Autodesk Fusion 360 part; units mm, degrees
note: some values were not read from the file. Set by a fixed rule: which sketch regions a step uses.
(part 4 of 6)
  spline S14 degree 5 poles (-6.3022, 4.9084) (-6.3022, 4.9084) (-6.3024, 4.9085) (-6.3026, 4.9086) (-6.3029, 4.9089) (-6.3033, 4.9092) (-6.3039, 4.9096) (-6.3045, 4.9101) (-6.3052, 4.9106) (-6.3059, 4.9111) (-6.3067, 4.9117) (-6.3076, 4.9124) (-6.3086, 4.913) (-6.3096, 4.9138) (-6.3107, 4.9145) (-6.3119, 4.9153) (-6.3131, 4.9162) (-6.3144, 4.9171) (-6.3158, 4.918) (-6.3173, 4.919) (-6.3188, 4.92) (-6.3203, 4.9211) (-6.322, 4.9221) (-6.3237, 4.9233) (-6.3254, 4.9244) (-6.3273, 4.9256) (-6.3292, 4.9268) (-6.3311, 4.9281) (-6.3332, 4.9294) (-6.3353, 4.9307) (-6.3374, 4.932) (-6.3396, 4.9334) (-6.3419, 4.9348) (-6.3443, 4.9363) (-6.3467, 4.9377) (-6.3491, 4.9392) (-6.3517, 4.9407) (-6.3543, 4.9423) (-6.3569, 4.9439) (-6.3596, 4.9454) (-6.3624, 4.9471) (-6.3652, 4.9487) (-6.3681, 4.9504) (-6.3711, 4.9521) (-6.3741, 4.9538) (-6.3772, 4.9555) (-6.3803, 4.9573) (-6.3835, 4.9591) (-6.3868, 4.9608) (-6.3901, 4.9627) (-6.3934, 4.9645) (-6.3969, 4.9664) (-6.4003, 4.9682) (-6.4039, 4.9701) (-6.4075, 4.972) (-6.4111, 4.9739) (-6.4149, 4.9759) (-6.4186, 4.9778) (-6.4224, 4.9798) (-6.4263, 4.9818) (-6.4303, 4.9838) (-6.4343, 4.9858) (-6.4383, 4.9878) (-6.4424, 4.9899) (-6.4466, 4.9919) (-6.4508, 4.994) (-6.455, 4.9961) (-6.4594, 4.9981) (-6.4637, 5.0002) (-6.4682, 5.0023) (-6.4727, 5.0045) (-6.4772, 5.0066) (-6.4818, 5.0087) (-6.4864, 5.0109) (-6.4911, 5.013) (-6.4959, 5.0152) (-6.5007, 5.0174) (-6.5055, 5.0195) (-6.5104, 5.0217) (-6.5154, 5.0239) (-6.5204, 5.0261) (-6.5255, 5.0283) (-6.5306, 5.0305) (-6.5357, 5.0327) (-6.541, 5.0349) (-6.5462, 5.0372) (-6.5515, 5.0394) (-6.5569, 5.0416) (-6.5623, 5.0439) (-6.5678, 5.0461) (-6.5733, 5.0483) (-6.5789, 5.0506) (-6.5845, 5.0528) (-6.5901, 5.0551) (-6.5959, 5.0573) (-6.6016, 5.0596) (-6.6074, 5.0618) (-6.6133, 5.0641) (-6.6192, 5.0664) (-6.6252, 5.0686) (-6.6312, 5.0709) (-6.6372, 5.0731) (-6.6433, 5.0754) (-6.6495, 5.0776) (-6.6556, 5.0799) (-6.6619, 5.0821) (-6.6682, 5.0844) (-6.6745, 5.0866) (-6.6809, 5.0889) (-6.6873, 5.0911) (-6.6938, 5.0933) (-6.7003, 5.0956) (-6.7069, 5.0978) (-6.7135, 5.1) (-6.7201, 5.1023) (-6.7269, 5.1045) (-6.7336, 5.1067) (-6.7404, 5.1089) (-6.7472, 5.1111) (-6.7541, 5.1133) (-6.761, 5.1155) (-6.768, 5.1177) (-6.775, 5.1199) (-6.7821, 5.1221) (-6.7892, 5.1242) (-6.7963, 5.1264) (-6.8035, 5.1286) (-6.8108, 5.1307) (-6.818, 5.1329) (-6.8254, 5.135) (-6.8327, 5.1371) (-6.8401, 5.1393) (-6.8476, 5.1414) (-6.8551, 5.1435) (-6.8626, 5.1456) (-6.8702, 5.1477) (-6.8778, 5.1498) (-6.8855, 5.1518) (-6.8932, 5.1539) (-6.9009, 5.1559) (-6.9087, 5.158) (-6.9165, 5.16) (-6.9244, 5.162) (-6.9323, 5.164) (-6.9403, 5.166) (-6.9483, 5.168) (-6.9563, 5.17) (-6.9644, 5.172) (-6.9725, 5.1739) (-6.9806, 5.1759) (-6.9888, 5.1778) (-6.997, 5.1797) (-7.0053, 5.1817) (-7.0136, 5.1836) (-7.022, 5.1854) (-7.0304, 5.1873) (-7.0388, 5.1892) (-7.0473, 5.191) (-7.0558, 5.1929) (-7.0643, 5.1947) (-7.0729, 5.1965) (-7.0815, 5.1983) (-7.0902, 5.2001) (-7.0989, 5.2018) (-7.1076, 5.2036) (-7.1164, 5.2053) (-7.1252, 5.207) (-7.1341, 5.2087) (-7.1429, 5.2104) (-7.1519, 5.2121) (-7.1608, 5.2138) (-7.1698, 5.2154) (-7.1789, 5.2171) (-7.1879, 5.2187) (-7.197, 5.2203) (-7.2062, 5.2219) (-7.2154, 5.2234) (-7.2246, 5.225) (-7.2338, 5.2265) (-7.2431, 5.228) (-7.2524, 5.2295) (-7.2618, 5.231) (-7.2712, 5.2325) (-7.2806, 5.2339) (-7.2901, 5.2354) (-7.2996, 5.2368) (-7.3091, 5.2382) (-7.3187, 5.2396) (-7.3283, 5.2409) (-7.3379, 5.2423) (-7.3476, 5.2436) (-7.3573, 5.2449) (-7.3671, 5.2462) (-7.3768, 5.2475) (-7.3866, 5.2487) (-7.3965, 5.25) (-7.4064, 5.2512) (-7.4163, 5.2524) (-7.4262, 5.2536) (-7.4362, 5.2547) (-7.4462, 5.2559) (-7.4562, 5.257) (-7.4663, 5.2581) (-7.4764, 5.2592) (-7.4865, 5.2602) (-7.4967, 5.2613) (-7.5069, 5.2623) (-7.5172, 5.2633) (-7.5274, 5.2642) (-7.5377, 5.2652) (-7.5481, 5.2661) (-7.5584, 5.2671) (-7.5688, 5.2679) (-7.5792, 5.2688) (-7.5897, 5.2697) (-7.6002, 5.2705) (-7.6107, 5.2713) (-7.6212, 5.2721) (-7.6318, 5.2729) (-7.6424, 5.2736) (-7.6531, 5.2743) (-7.6637, 5.275) (-7.6744, 5.2757) (-7.6852, 5.2764) (-7.6959, 5.277) (-7.7067, 5.2776) (-7.7175, 5.2782) (-7.7284, 5.2788) (-7.7393, 5.2793) (-7.7502, 5.2798) (-7.7611, 5.2803) (-7.7721, 5.2808) (-7.7831, 5.2813) (-7.7941, 5.2817) (-7.8052, 5.2821) (-7.8162, 5.2825) (-7.8273, 5.2828) (-7.8385, 5.2832) (-7.8496, 5.2835) (-7.8608, 5.2837) (-7.8721, 5.284) (-7.8811, 5.2842) (-7.8878, 5.2843) (-7.8923, 5.2844) (-7.8946, 5.2845) knots 0 0 0 0 0 0 0.00416667 0.00833333 0.0125 0.01666667 0.02083333 0.025 0.02916667 0.03333333 0.0375 0.04166667 0.04583333 0.05 0.05416667 0.05833333 0.0625 0.06666667 0.07083333 0.075 0.07916667 0.08333333 0.0875 0.09166667 0.09583333 0.1 0.10416667 0.10833333 0.1125 0.11666667 0.12083333 0.125 0.12916667 0.13333333 0.1375 0.14166667 0.14583333 0.15 0.15416667 0.15833333 0.1625 0.16666667 0.17083333 0.175 0.17916667 0.18333333 0.1875 0.19166667 0.19583333 0.2 0.20416667 0.20833333 0.2125 0.21666667 0.22083333 0.225 0.22916667 0.23333333 0.2375 0.24166667 0.24583333 0.25 0.25416667 0.25833333 0.2625 0.26666667 0.27083333 0.275 0.27916667 0.28333333 0.2875 0.29166667 0.29583333 0.3 0.30416667 0.30833333 0.3125 0.31666667 0.32083333 0.325 0.32916667 0.33333333 0.3375 0.34166667 0.34583333 0.35 0.35416667 0.35833333 0.3625 0.36666667 0.37083333 0.375 0.37916667 0.38333333 0.3875 0.39166667 0.39583333 0.4 0.40416667 0.40833333 0.4125 0.41666667 0.42083333 0.425 0.42916667 0.43333333 0.4375 0.44166667 0.44583333 0.45 0.45416667 0.45833333 0.4625 0.46666667 0.47083333 0.475 0.47916667 0.48333333 0.4875 0.49166667 0.49583333 0.5 0.50416667 0.50833333 0.5125 0.51666667 0.52083333 0.525 0.52916667 0.53333333 0.5375 0.54166667 0.54583333 0.55 0.55416667 0.55833333 0.5625 0.56666667 0.57083333 0.575 0.57916667 0.58333333 0.5875 0.59166667 0.59583333 0.6 0.60416667 0.60833333 0.6125 0.61666667 0.62083333 0.625 0.62916667 0.63333333 0.6375 0.64166667 0.64583333 0.65 0.65416667 0.65833333 0.6625 0.66666667 0.67083333 0.675 0.67916667 0.68333333 0.6875 0.69166667 0.69583333 0.7 0.70416667 0.70833333 0.7125 0.71666667 0.72083333 0.725 0.72916667 0.73333333 0.7375 0.74166667 0.74583333 0.75 0.75416667 0.75833333 0.7625 0.76666667 0.77083333 0.775 0.77916667 0.78333333 0.7875 0.79166667 0.79583333 0.8 0.80416667 0.80833333 0.8125 0.81666667 0.82083333 0.825 0.82916667 0.83333333 0.8375 0.84166667 0.84583333 0.85 0.85416667 0.85833333 0.8625 0.86666667 0.87083333 0.875 0.87916667 0.88333333 0.8875 0.89166667 0.89583333 0.9 0.90416667 0.90833333 0.9125 0.91666667 0.92083333 0.925 0.92916667 0.93333333 0.9375 0.94166667 0.94583333 0.95 0.95416667 0.95833333 0.9625 0.96666667 0.97083333 0.975 0.97916667 0.98333333 0.9875 0.99166667 0.99583333 1 1 1 1 1 1
  arc A15 (-7.8946, 5.2845) -> (-8.2494, 4.7115) centre (0, 0) ccw
  spline S15 degree 5 poles (-8.2494, 4.7115) (-8.2483, 4.7095) (-8.2462, 4.7055) (-8.2431, 4.6995) (-8.2389, 4.6915) (-8.2337, 4.6816) (-8.2284, 4.6717) (-8.2232, 4.6618) (-8.2179, 4.652) (-8.2127, 4.6422) (-8.2074, 4.6325) (-8.2021, 4.6227) (-8.1968, 4.6131) (-8.1915, 4.6034) (-8.1862, 4.5938) (-8.1809, 4.5843) (-8.1755, 4.5747) (-8.1702, 4.5652) (-8.1649, 4.5558) (-8.1595, 4.5463) (-8.1542, 4.537) (-8.1488, 4.5276) (-8.1434, 4.5183) (-8.138, 4.509) (-8.1327, 4.4998) (-8.1273, 4.4906) (-8.1219, 4.4814) (-8.1165, 4.4723) (-8.1111, 4.4632) (-8.1057, 4.4541) (-8.1002, 4.4451) (-8.0948, 4.4361) (-8.0894, 4.4272) (-8.084, 4.4183) (-8.0785, 4.4094) (-8.0731, 4.4006) (-8.0676, 4.3918) (-8.0622, 4.383) (-8.0567, 4.3743) (-8.0513, 4.3656) (-8.0458, 4.357) (-8.0403, 4.3484) (-8.0349, 4.3398) (-8.0294, 4.3313) (-8.0239, 4.3228) (-8.0184, 4.3144) (-8.0129, 4.306) (-8.0075, 4.2976) (-8.002, 4.2892) (-7.9965, 4.2809) (-7.991, 4.2727) (-7.9855, 4.2645) (-7.98, 4.2563) (-7.9745, 4.2481) (-7.969, 4.24) (-7.9635, 4.232) (-7.958, 4.2239) (-7.9525, 4.2159) (-7.947, 4.208) (-7.9415, 4.2001) (-7.936, 4.1922) (-7.9305, 4.1844) (-7.925, 4.1766) (-7.9195, 4.1688) (-7.914, 4.1611) (-7.9085, 4.1534) (-7.903, 4.1458) (-7.8975, 4.1382) (-7.892, 4.1306) (-7.8865, 4.1231) (-7.881, 4.1156) (-7.8755, 4.1082) (-7.87, 4.1008) (-7.8645, 4.0934) (-7.859, 4.0861) (-7.8536, 4.0788) (-7.8481, 4.0716) (-7.8426, 4.0644) (-7.8371, 4.0572) (-7.8317, 4.0501) (-7.8262, 4.043) (-7.8207, 4.036) (-7.8153, 4.029) (-7.8098, 4.022) (-7.8044, 4.0151) (-7.7989, 4.0082) (-7.7935, 4.0014) (-7.788, 3.9946) (-7.7826, 3.9879) (-7.7772, 3.9811) (-7.7718, 3.9745) (-7.7664, 3.9678) (-7.761, 3.9612) (-7.7556, 3.9547) (-7.7502, 3.9482) (-7.7448, 3.9417) (-7.7394, 3.9353) (-7.7341, 3.9289) (-7.7287, 3.9225) (-7.7233, 3.9162) (-7.718, 3.91) (-7.7127, 3.9037) (-7.7073, 3.8976) (-7.702, 3.8914) (-7.6967, 3.8853) (-7.6914, 3.8793) (-7.6861, 3.8732) (-7.6808, 3.8673) (-7.6756, 3.8613) (-7.6703, 3.8554) (-7.6651, 3.8496) (-7.6598, 3.8438) (-7.6546, 3.838) (-7.6494, 3.8323) (-7.6442, 3.8266) (-7.639, 3.8209) (-7.6338, 3.8153) (-7.6287, 3.8098) (-7.6235, 3.8043) (-7.6184, 3.7988) (-7.6132, 3.7934) (-7.6081, 3.788) (-7.603, 3.7826) (-7.5979, 3.7773) (-7.5929, 3.7721) (-7.5878, 3.7668) (-7.5828, 3.7616) (-7.5778, 3.7565) (-7.5728, 3.7514) (-7.5678, 3.7464) (-7.5628, 3.7414) (-7.5578, 3.7364) (-7.5529, 3.7315) (-7.548, 3.7266) (-7.5431, 3.7217) (-7.5382, 3.7169) (-7.5333, 3.7122) (-7.5284, 3.7075) (-7.5236, 3.7028) (-7.5188, 3.6982) (-7.514, 3.6936) (-7.5092, 3.6891) (-7.5045, 3.6846) (-7.4997, 3.6801) (-7.495, 3.6757) (-7.4903, 3.6713) (-7.4856, 3.667) (-7.481, 3.6627) (-7.4764, 3.6585) (-7.4718, 3.6543) (-7.4672, 3.6501) (-7.4626, 3.646) (-7.4581, 3.6419) (-7.4536, 3.6379) (-7.4491, 3.6339) (-7.4446, 3.63) (-7.4402, 3.6261) (-7.4357, 3.6222) (-7.4314, 3.6184) (-7.427, 3.6147) (-7.4227, 3.611) (-7.4183, 3.6073) (-7.4141, 3.6036) (-7.4098, 3.6) (-7.4056, 3.5965) (-7.4014, 3.593) (-7.3972, 3.5895) (-7.3931, 3.5861) (-7.389, 3.5827) (-7.3849, 3.5794) (-7.3808, 3.5761) (-7.3768, 3.5729) (-7.3728, 3.5697) (-7.3688, 3.5665) (-7.3649, 3.5634) (-7.361, 3.5603) (-7.3572, 3.5573) (-7.3533, 3.5543) (-7.3495, 3.5514) (-7.3458, 3.5485) (-7.3421, 3.5456) (-7.3384, 3.5428) (-7.3347, 3.5401) (-7.3311, 3.5374) (-7.3275, 3.5347) (-7.324, 3.532) (-7.3205, 3.5295) (-7.317, 3.5269) (-7.3136, 3.5244) (-7.3102, 3.5219) (-7.3068, 3.5195) (-7.3035, 3.5172) (-7.3003, 3.5148) (-7.297, 3.5125) (-7.2938, 3.5103) (-7.2907, 3.5081) (-7.2876, 3.506) (-7.2845, 3.5038) (-7.2815, 3.5018) (-7.2786, 3.4998) (-7.2756, 3.4978) (-7.2728, 3.4958) (-7.2699, 3.4939) (-7.2671, 3.4921) (-7.2644, 3.4903) (-7.2617, 3.4885) (-7.2591, 3.4868) (-7.2565, 3.4851) (-7.2539, 3.4835) (-7.2515, 3.4819) (-7.249, 3.4804) (-7.2466, 3.4789) (-7.2443, 3.4774) (-7.242, 3.476) (-7.2398, 3.4746) (-7.2376, 3.4733) (-7.2355, 3.472) (-7.2335, 3.4708) (-7.2315, 3.4696) (-7.2295, 3.4684) (-7.2276, 3.4673) (-7.2258, 3.4662) (-7.2241, 3.4652) (-7.2224, 3.4642) (-7.2207, 3.4633) (-7.2191, 3.4624) (-7.2176, 3.4615) (-7.2162, 3.4607) (-7.2148, 3.46) (-7.2135, 3.4592) (-7.2122, 3.4585) (-7.2111, 3.4579) (-7.21, 3.4573) (-7.2089, 3.4567) (-7.2079, 3.4562) (-7.207, 3.4558) (-7.2062, 3.4553) (-7.2055, 3.4549) (-7.2048, 3.4546) (-7.2042, 3.4543) (-7.2037, 3.454) (-7.2033, 3.4538) (-7.2031, 3.4537) (-7.203, 3.4537) (-7.2029, 3.4536) knots -1 -1 -1 -1 -1 -1 -0.99583333 -0.99166667 -0.9875 -0.98333333 -0.97916667 -0.975 -0.97083333 -0.96666667 -0.9625 -0.95833333 -0.95416667 -0.95 -0.94583333 -0.94166667 -0.9375 -0.93333333 -0.92916667 -0.925 -0.92083333 -0.91666667 -0.9125 -0.90833333 -0.90416667 -0.9 -0.89583333 -0.89166667 -0.8875 -0.88333333 -0.87916667 -0.875 -0.87083333 -0.86666667 -0.8625 -0.85833333 -0.85416667 -0.85 -0.84583333 -0.84166667 -0.8375 -0.83333333 -0.82916667 -0.825 -0.82083333 -0.81666667 -0.8125 -0.80833333 -0.80416667 -0.8 -0.79583333 -0.79166667 -0.7875 -0.78333333 -0.77916667 -0.775 -0.77083333 -0.76666667 -0.7625 -0.75833333 -0.75416667 -0.75 -0.74583333 -0.74166667 -0.7375 -0.73333333 -0.72916667 -0.725 -0.72083333 -0.71666667 -0.7125 -0.70833333 -0.70416667 -0.7 -0.69583333 -0.69166667 -0.6875 -0.68333333 -0.67916667 -0.675 -0.67083333 -0.66666667 -0.6625 -0.65833333 -0.65416667 -0.65 -0.64583333 -0.64166667 -0.6375 -0.63333333 -0.62916667 -0.625 -0.62083333 -0.61666667 -0.6125 -0.60833333 -0.60416667 -0.6 -0.59583333 -0.59166667 -0.5875 -0.58333333 -0.57916667 -0.575 -0.57083333 -0.56666667 -0.5625 -0.55833333 -0.55416667 -0.55 -0.54583333 -0.54166667 -0.5375 -0.53333333 -0.52916667 -0.525 -0.52083333 -0.51666667 -0.5125 -0.50833333 -0.50416667 -0.5 -0.49583333 -0.49166667 -0.4875 -0.48333333 -0.47916667 -0.475 -0.47083333 -0.46666667 -0.4625 -0.45833333 -0.45416667 -0.45 -0.44583333 -0.44166667 -0.4375 -0.43333333 -0.42916667 -0.425 -0.42083333 -0.41666667 -0.4125 -0.40833333 -0.40416667 -0.4 -0.39583333 -0.39166667 -0.3875 -0.38333333 -0.37916667 -0.375 -0.37083333 -0.36666667 -0.3625 -0.35833333 -0.35416667 -0.35 -0.34583333 -0.34166667 -0.3375 -0.33333333 -0.32916667 -0.325 -0.32083333 -0.31666667 -0.3125 -0.30833333 -0.30416667 -0.3 -0.29583333 -0.29166667 -0.2875 -0.28333333 -0.27916667 -0.275 -0.27083333 -0.26666667 -0.2625 -0.25833333 -0.25416667 -0.25 -0.24583333 -0.24166667 -0.2375 -0.23333333 -0.22916667 -0.225 -0.22083333 -0.21666667 -0.2125 -0.20833333 -0.20416667 -0.2 -0.19583333 -0.19166667 -0.1875 -0.18333333 -0.17916667 -0.175 -0.17083333 -0.16666667 -0.1625 -0.15833333 -0.15416667 -0.15 -0.14583333 -0.14166667 -0.1375 -0.13333333 -0.12916667 -0.125 -0.12083333 -0.11666667 -0.1125 -0.10833333 -0.10416667 -0.1 -0.09583333 -0.09166667 -0.0875 -0.08333333 -0.07916667 -0.075 -0.07083333 -0.06666667 -0.0625 -0.05833333 -0.05416667 -0.05 -0.04583333 -0.04166667 -0.0375 -0.03333333 -0.02916667 -0.025 -0.02083333 -0.01666667 -0.0125 -0.00833333 -0.00416667 0 0 0 0 0 0
  line L30 (-7.2029, 3.4536) -> (-7.2023, 3.4533)
  line L31 (-7.2023, 3.4533) -> (-6.5374, 3.1345)
  arc A16 (-6.5374, 3.1345) -> (-6.9429, 2.0878) centre (0, 0) ccw
  line L32 (-6.9429, 2.0878) -> (-7.649, 2.3001)
  line L33 (-7.649, 2.3001) -> (-7.6497, 2.3003)
  spline S16 degree 5 poles (-7.6497, 2.3003) (-7.6498, 2.3003) (-7.6499, 2.3004) (-7.6502, 2.3004) (-7.6505, 2.3005) (-7.6511, 2.3007) (-7.6518, 2.3009) (-7.6525, 2.3011) (-7.6533, 2.3013) (-7.6542, 2.3015) (-7.6552, 2.3018) (-7.6562, 2.302) (-7.6574, 2.3023) (-7.6586, 2.3026) (-7.6599, 2.303) (-7.6613, 2.3033) (-7.6628, 2.3036) (-7.6643, 2.304) (-7.6659, 2.3044) (-7.6676, 2.3048) (-7.6694, 2.3052) (-7.6712, 2.3056) (-7.6731, 2.306) (-7.6751, 2.3064) (-7.6772, 2.3069) (-7.6793, 2.3073) (-7.6816, 2.3078) (-7.6838, 2.3082) (-7.6862, 2.3087) (-7.6886, 2.3092) (-7.6911, 2.3096) (-7.6937, 2.3101) (-7.6963, 2.3106) (-7.699, 2.3111) (-7.7018, 2.3116) (-7.7046, 2.3121) (-7.7076, 2.3126) (-7.7105, 2.3131) (-7.7136, 2.3136) (-7.7167, 2.3141) (-7.7199, 2.3146) (-7.7231, 2.3151) (-7.7264, 2.3157) (-7.7298, 2.3162) (-7.7332, 2.3167) (-7.7367, 2.3172) (-7.7402, 2.3177) (-7.7439, 2.3182) (-7.7475, 2.3187) (-7.7513, 2.3192) (-7.7551, 2.3197) (-7.759, 2.3202) (-7.7629, 2.3207) (-7.7669, 2.3211) (-7.7709, 2.3216) (-7.775, 2.3221) (-7.7792, 2.3226) (-7.7834, 2.323) (-7.7877, 2.3235) (-7.792, 2.3239) (-7.7964, 2.3244) (-7.8008, 2.3248) (-7.8054, 2.3252) (-7.8099, 2.3256) (-7.8145, 2.3261) (-7.8192, 2.3265) (-7.8239, 2.3268) (-7.8287, 2.3272) (-7.8336, 2.3276) (-7.8384, 2.328) (-7.8434, 2.3283) (-7.8484, 2.3287) (-7.8534, 2.329) (-7.8586, 2.3293) (-7.8637, 2.3296) (-7.8689, 2.3299) (-7.8742, 2.3302) (-7.8795, 2.3305) (-7.8849, 2.3308) (-7.8903, 2.331) (-7.8957, 2.3313) (-7.9012, 2.3315) (-7.9068, 2.3317) (-7.9124, 2.3319) (-7.9181, 2.3321) (-7.9238, 2.3323) (-7.9296, 2.3324) (-7.9354, 2.3326) (-7.9412, 2.3327) (-7.9471, 2.3328) (-7.9531, 2.3329) (-7.9591, 2.333) (-7.9651, 2.333) (-7.9712, 2.3331) (-7.9774, 2.3331) (-7.9836, 2.3331) (-7.9898, 2.3331) (-7.9961, 2.3331) (-8.0024, 2.3331) (-8.0088, 2.3331) (-8.0152, 2.333) (-8.0216, 2.3329) (-8.0281, 2.3328) (-8.0347, 2.3327) (-8.0413, 2.3325) (-8.0479, 2.3324) (-8.0546, 2.3322) (-8.0613, 2.332) (-8.0681, 2.3318) (-8.0749, 2.3316) (-8.0817, 2.3313) (-8.0886, 2.3311) (-8.0955, 2.3308) (-8.1025, 2.3305) (-8.1095, 2.3301) (-8.1166, 2.3298) (-8.1236, 2.3294) (-8.1308, 2.329) (-8.138, 2.3286) (-8.1452, 2.3282) (-8.1524, 2.3277) (-8.1597, 2.3272) (-8.167, 2.3267) (-8.1744, 2.3262) (-8.1818, 2.3257) (-8.1893, 2.3251) (-8.1968, 2.3245) (-8.2043, 2.3239) (-8.2118, 2.3233) (-8.2194, 2.3226) (-8.2271, 2.322) (-8.2348, 2.3213) (-8.2425, 2.3206) (-8.2502, 2.3198) (-8.258, 2.3191) (-8.2658, 2.3183) (-8.2737, 2.3174) (-8.2816, 2.3166) (-8.2895, 2.3158) (-8.2975, 2.3149) (-8.3055, 2.314) (-8.3135, 2.313) (-8.3216, 2.3121) (-8.3297, 2.3111) (-8.3378, 2.3101) (-8.346, 2.3091) (-8.3542, 2.308) (-8.3624, 2.3069) (-8.3707, 2.3058) (-8.379, 2.3047) (-8.3873, 2.3035) (-8.3957, 2.3023) (-8.4041, 2.3011) (-8.4125, 2.2999) (-8.421, 2.2986) (-8.4295, 2.2974) (-8.438, 2.2961) (-8.4466, 2.2947) (-8.4552, 2.2934) (-8.4638, 2.292) (-8.4725, 2.2906) (-8.4812, 2.2891) (-8.4899, 2.2876) (-8.4986, 2.2861) (-8.5074, 2.2846) (-8.5162, 2.2831) (-8.5251, 2.2815) (-8.5339, 2.2799) (-8.5428, 2.2783) (-8.5517, 2.2766) (-8.5607, 2.2749) (-8.5697, 2.2732) (-8.5787, 2.2715) (-8.5877, 2.2697) (-8.5968, 2.2679) (-8.6059, 2.2661) (-8.615, 2.2642) (-8.6242, 2.2623) (-8.6334, 2.2604) (-8.6426, 2.2585) (-8.6518, 2.2565) (-8.6611, 2.2545) (-8.6704, 2.2525) (-8.6797, 2.2504) (-8.689, 2.2484) (-8.6984, 2.2463) (-8.7078, 2.2441) (-8.7172, 2.2419) (-8.7267, 2.2397) (-8.7361, 2.2375) (-8.7456, 2.2353) (-8.7552, 2.233) (-8.7647, 2.2307) (-8.7743, 2.2283) (-8.7839, 2.2259) (-8.7935, 2.2235) (-8.8032, 2.2211) (-8.8128, 2.2186) (-8.8225, 2.2161) (-8.8323, 2.2136) (-8.842, 2.2111) (-8.8518, 2.2085) (-8.8616, 2.2059) (-8.8714, 2.2032) (-8.8812, 2.2005) (-8.8911, 2.1978) (-8.9009, 2.1951) (-8.9109, 2.1923) (-8.9208, 2.1895) (-8.9307, 2.1867) (-8.9407, 2.1839) (-8.9507, 2.181) (-8.9607, 2.178) (-8.9707, 2.1751) (-8.9808, 2.1721) (-8.9909, 2.1691) (-9.001, 2.1661) (-9.0111, 2.163) (-9.0212, 2.1599) (-9.0314, 2.1567) (-9.0416, 2.1536) (-9.0518, 2.1504) (-9.062, 2.1471) (-9.0723, 2.1439) (-9.0825, 2.1406) (-9.0928, 2.1372) (-9.1031, 2.1339) (-9.1134, 2.1305) (-9.1238, 2.1271) (-9.1341, 2.1236) (-9.1445, 2.1201) (-9.1549, 2.1166) (-9.1653, 2.113) (-9.1757, 2.1095) (-9.1862, 2.1058) (-9.1967, 2.1022) (-9.2072, 2.0985) (-9.2177, 2.0948) (-9.2282, 2.0911) (-9.2387, 2.0873) (-9.2493, 2.0835) (-9.2577, 2.0804) (-9.2641, 2.0781) (-9.2683, 2.0765) (-9.2705, 2.0758) knots 0 0 0 0 0 0 0.00416667 0.00833333 0.0125 0.01666667 0.02083333 0.025 0.02916667 0.03333333 0.0375 0.04166667 0.04583333 0.05 0.05416667 0.05833333 0.0625 0.06666667 0.07083333 0.075 0.07916667 0.08333333 0.0875 0.09166667 0.09583333 0.1 0.10416667 0.10833333 0.1125 0.11666667 0.12083333 0.125 0.12916667 0.13333333 0.1375 0.14166667 0.14583333 0.15 0.15416667 0.15833333 0.1625 0.16666667 0.17083333 0.175 0.17916667 0.18333333 0.1875 0.19166667 0.19583333 0.2 0.20416667 0.20833333 0.2125 0.21666667 0.22083333 0.225 0.22916667 0.23333333 0.2375 0.24166667 0.24583333 0.25 0.25416667 0.25833333 0.2625 0.26666667 0.27083333 0.275 0.27916667 0.28333333 0.2875 0.29166667 0.29583333 0.3 0.30416667 0.30833333 0.3125 0.31666667 0.32083333 0.325 0.32916667 0.33333333 0.3375 0.34166667 0.34583333 0.35 0.35416667 0.35833333 0.3625 0.36666667 0.37083333 0.375 0.37916667 0.38333333 0.3875 0.39166667 0.39583333 0.4 0.40416667 0.40833333 0.4125 0.41666667 0.42083333 0.425 0.42916667 0.43333333 0.4375 0.44166667 0.44583333 0.45 0.45416667 0.45833333 0.4625 0.46666667 0.47083333 0.475 0.47916667 0.48333333 0.4875 0.49166667 0.49583333 0.5 0.50416667 0.50833333 0.5125 0.51666667 0.52083333 0.525 0.52916667 0.53333333 0.5375 0.54166667 0.54583333 0.55 0.55416667 0.55833333 0.5625 0.56666667 0.57083333 0.575 0.57916667 0.58333333 0.5875 0.59166667 0.59583333 0.6 0.60416667 0.60833333 0.6125 0.61666667 0.62083333 0.625 0.62916667 0.63333333 0.6375 0.64166667 0.64583333 0.65 0.65416667 0.65833333 0.6625 0.66666667 0.67083333 0.675 0.67916667 0.68333333 0.6875 0.69166667 0.69583333 0.7 0.70416667 0.70833333 0.7125 0.71666667 0.72083333 0.725 0.72916667 0.73333333 0.7375 0.74166667 0.74583333 0.75 0.75416667 0.75833333 0.7625 0.76666667 0.77083333 0.775 0.77916667 0.78333333 0.7875 0.79166667 0.79583333 0.8 0.80416667 0.80833333 0.8125 0.81666667 0.82083333 0.825 0.82916667 0.83333333 0.8375 0.84166667 0.84583333 0.85 0.85416667 0.85833333 0.8625 0.86666667 0.87083333 0.875 0.87916667 0.88333333 0.8875 0.89166667 0.89583333 0.9 0.90416667 0.90833333 0.9125 0.91666667 0.92083333 0.925 0.92916667 0.93333333 0.9375 0.94166667 0.94583333 0.95 0.95416667 0.95833333 0.9625 0.96666667 0.97083333 0.975 0.97916667 0.98333333 0.9875 0.99166667 0.99583333 1 1 1 1 1 1
  arc A17 (-9.2705, 2.0758) -> (-9.3943, 1.4133) centre (0, 0) ccw
  spline S17 degree 5 poles (-9.3943, 1.4133) (-9.3926, 1.4118) (-9.3892, 1.4088) (-9.3841, 1.4044) (-9.3773, 1.3984) (-9.3689, 1.3911) (-9.3604, 1.3837) (-9.3519, 1.3765) (-9.3435, 1.3692) (-9.335, 1.362) (-9.3266, 1.3548) (-9.3182, 1.3476) (-9.3097, 1.3405) (-9.3013, 1.3335) (-9.2929, 1.3264) (-9.2845, 1.3194) (-9.276, 1.3125) (-9.2676, 1.3055) (-9.2592, 1.2986) (-9.2508, 1.2918) (-9.2425, 1.285) (-9.2341, 1.2782) (-9.2257, 1.2714) (-9.2173, 1.2647) (-9.209, 1.2581) (-9.2006, 1.2514) (-9.1923, 1.2448) (-9.184, 1.2383) (-9.1756, 1.2317) (-9.1673, 1.2253) (-9.159, 1.2188) (-9.1507, 1.2124) (-9.1424, 1.206) (-9.1341, 1.1997) (-9.1259, 1.1934) (-9.1176, 1.1871) (-9.1093, 1.1809) (-9.1011, 1.1747) (-9.0929, 1.1685) (-9.0846, 1.1624) (-9.0764, 1.1563) (-9.0682, 1.1503) (-9.06, 1.1443) (-9.0518, 1.1383) (-9.0436, 1.1323) (-9.0355, 1.1264) (-9.0273, 1.1206) (-9.0192, 1.1147) (-9.0111, 1.109) (-9.0029, 1.1032) (-8.9948, 1.0975) (-8.9867, 1.0918) (-8.9787, 1.0862) (-8.9706, 1.0805) (-8.9625, 1.075) (-8.9545, 1.0694) (-8.9465, 1.0639) (-8.9385, 1.0585) (-8.9305, 1.0531) (-8.9225, 1.0477) (-8.9145, 1.0423) (-8.9065, 1.037) (-8.8986, 1.0317) (-8.8906, 1.0265) (-8.8827, 1.0213) (-8.8748, 1.0161) (-8.8669, 1.011) (-8.8591, 1.0059) (-8.8512, 1.0008) (-8.8434, 0.9958) (-8.8355, 0.9908) (-8.8277, 0.9858) (-8.8199, 0.9809) (-8.8122, 0.976) (-8.8044, 0.9712) (-8.7967, 0.9664) (-8.7889, 0.9616) (-8.7812, 0.9569) (-8.7735, 0.9522) (-8.7659, 0.9475) (-8.7582, 0.9429) (-8.7506, 0.9383) (-8.743, 0.9337) (-8.7354, 0.9292) (-8.7278, 0.9247) (-8.7202, 0.9203) (-8.7127, 0.9159) (-8.7052, 0.9115) (-8.6977, 0.9072) (-8.6902, 0.9029) (-8.6827, 0.8986) (-8.6753, 0.8944) (-8.6679, 0.8902) (-8.6605, 0.886) (-8.6531, 0.8819) (-8.6457, 0.8778) (-8.6384, 0.8737) (-8.6311, 0.8697) (-8.6238, 0.8657) (-8.6165, 0.8618) (-8.6093, 0.8579) (-8.602, 0.854) (-8.5948, 0.8501) (-8.5877, 0.8463) (-8.5805, 0.8426) (-8.5734, 0.8388) (-8.5663, 0.8351) (-8.5592, 0.8315) (-8.5521, 0.8278) (-8.5451, 0.8242) (-8.5381, 0.8207) (-8.5311, 0.8172) (-8.5242, 0.8137) (-8.5172, 0.8102) (-8.5103, 0.8068) (-8.5034, 0.8034) (-8.4966, 0.8) (-8.4898, 0.7967) (-8.483, 0.7934) (-8.4762, 0.7902) (-8.4695, 0.787) (-8.4627, 0.7838) (-8.4561, 0.7807) (-8.4494, 0.7775) (-8.4428, 0.7745) (-8.4362, 0.7714) (-8.4296, 0.7684) (-8.4231, 0.7654) (-8.4166, 0.7625) (-8.4101, 0.7596) (-8.4036, 0.7567) (-8.3972, 0.7539) (-8.3908, 0.7511) (-8.3845, 0.7483) (-8.3781, 0.7456) (-8.3718, 0.7428) (-8.3656, 0.7402) (-8.3594, 0.7375) (-8.3532, 0.7349) (-8.347, 0.7324) (-8.3409, 0.7298) (-8.3348, 0.7273) (-8.3287, 0.7248) (-8.3227, 0.7224) (-8.3167, 0.72) (-8.3107, 0.7176) (-8.3048, 0.7152) (-8.2989, 0.7129) (-8.2931, 0.7106) (-8.2873, 0.7084) (-8.2815, 0.7062) (-8.2758, 0.704) (-8.2701, 0.7018) (-8.2644, 0.6997) (-8.2588, 0.6976) (-8.2532, 0.6956) (-8.2476, 0.6935) (-8.2421, 0.6915) (-8.2367, 0.6896) (-8.2312, 0.6876) (-8.2258, 0.6857) (-8.2205, 0.6839) (-8.2152, 0.682) (-8.2099, 0.6802) (-8.2047, 0.6784) (-8.1995, 0.6767) (-8.1944, 0.675) (-8.1893, 0.6733) (-8.1842, 0.6716) (-8.1792, 0.67) (-8.1743, 0.6684) (-8.1693, 0.6668) (-8.1645, 0.6653) (-8.1596, 0.6637) (-8.1548, 0.6623) (-8.1501, 0.6608) (-8.1454, 0.6594) (-8.1408, 0.658) (-8.1362, 0.6566) (-8.1316, 0.6553) (-8.1271, 0.654) (-8.1226, 0.6527) (-8.1182, 0.6514) (-8.1139, 0.6502) (-8.1096, 0.649) (-8.1053, 0.6478) (-8.1011, 0.6467) (-8.097, 0.6455) (-8.0929, 0.6444) (-8.0888, 0.6434) (-8.0848, 0.6423) (-8.0809, 0.6413) (-8.077, 0.6403) (-8.0732, 0.6394) (-8.0694, 0.6384) (-8.0656, 0.6375) (-8.062, 0.6366) (-8.0584, 0.6358) (-8.0548, 0.6349) (-8.0513, 0.6341) (-8.0479, 0.6333) (-8.0445, 0.6325) (-8.0412, 0.6318) (-8.0379, 0.6311) (-8.0347, 0.6304) (-8.0316, 0.6297) (-8.0285, 0.6291) (-8.0254, 0.6284) (-8.0225, 0.6278) (-8.0196, 0.6273) (-8.0168, 0.6267) (-8.014, 0.6262) (-8.0113, 0.6256) (-8.0087, 0.6252) (-8.0061, 0.6247) (-8.0036, 0.6242) (-8.0012, 0.6238) (-7.9988, 0.6234) (-7.9965, 0.623) (-7.9943, 0.6226) (-7.9921, 0.6222) (-7.99, 0.6219) (-7.988, 0.6216) (-7.9861, 0.6213) (-7.9842, 0.621) (-7.9824, 0.6207) (-7.9807, 0.6205) (-7.979, 0.6202) (-7.9775, 0.62) (-7.976, 0.6198) (-7.9746, 0.6196) (-7.9733, 0.6195) (-7.972, 0.6193) (-7.9708, 0.6192) (-7.9697, 0.619) (-7.9687, 0.6189) (-7.9678, 0.6188) (-7.967, 0.6187) (-7.9662, 0.6186) (-7.9656, 0.6186) (-7.965, 0.6185) (-7.9646, 0.6185) (-7.9643, 0.6184) (-7.9642, 0.6184) (-7.9641, 0.6184) knots -1 -1 -1 -1 -1 -1 -0.99583333 -0.99166667 -0.9875 -0.98333333 -0.97916667 -0.975 -0.97083333 -0.96666667 -0.9625 -0.95833333 -0.95416667 -0.95 -0.94583333 -0.94166667 -0.9375 -0.93333333 -0.92916667 -0.925 -0.92083333 -0.91666667 -0.9125 -0.90833333 -0.90416667 -0.9 -0.89583333 -0.89166667 -0.8875 -0.88333333 -0.87916667 -0.875 -0.87083333 -0.86666667 -0.8625 -0.85833333 -0.85416667 -0.85 -0.84583333 -0.84166667 -0.8375 -0.83333333 -0.82916667 -0.825 -0.82083333 -0.81666667 -0.8125 -0.80833333 -0.80416667 -0.8 -0.79583333 -0.79166667 -0.7875 -0.78333333 -0.77916667 -0.775 -0.77083333 -0.76666667 -0.7625 -0.75833333 -0.75416667 -0.75 -0.74583333 -0.74166667 -0.7375 -0.73333333 -0.72916667 -0.725 -0.72083333 -0.71666667 -0.7125 -0.70833333 -0.70416667 -0.7 -0.69583333 -0.69166667 -0.6875 -0.68333333 -0.67916667 -0.675 -0.67083333 -0.66666667 -0.6625 -0.65833333 -0.65416667 -0.65 -0.64583333 -0.64166667 -0.6375 -0.63333333 -0.62916667 -0.625 -0.62083333 -0.61666667 -0.6125 -0.60833333 -0.60416667 -0.6 -0.59583333 -0.59166667 -0.5875 -0.58333333 -0.57916667 -0.575 -0.57083333 -0.56666667 -0.5625 -0.55833333 -0.55416667 -0.55 -0.54583333 -0.54166667 -0.5375 -0.53333333 -0.52916667 -0.525 -0.52083333 -0.51666667 -0.5125 -0.50833333 -0.50416667 -0.5 -0.49583333 -0.49166667 -0.4875 -0.48333333 -0.47916667 -0.475 -0.47083333 -0.46666667 -0.4625 -0.45833333 -0.45416667 -0.45 -0.44583333 -0.44166667 -0.4375 -0.43333333 -0.42916667 -0.425 -0.42083333 -0.41666667 -0.4125 -0.40833333 -0.40416667 -0.4 -0.39583333 -0.39166667 -0.3875 -0.38333333 -0.37916667 -0.375 -0.37083333 -0.36666667 -0.3625 -0.35833333 -0.35416667 -0.35 -0.34583333 -0.34166667 -0.3375 -0.33333333 -0.32916667 -0.325 -0.32083333 -0.31666667 -0.3125 -0.30833333 -0.30416667 -0.3 -0.29583333 -0.29166667 -0.2875 -0.28333333 -0.27916667 -0.275 -0.27083333 -0.26666667 -0.2625 -0.25833333 -0.25416667 -0.25 -0.24583333 -0.24166667 -0.2375 -0.23333333 -0.22916667 -0.225 -0.22083333 -0.21666667 -0.2125 -0.20833333 -0.20416667 -0.2 -0.19583333 -0.19166667 -0.1875 -0.18333333 -0.17916667 -0.175 -0.17083333 -0.16666667 -0.1625 -0.15833333 -0.15416667 -0.15 -0.14583333 -0.14166667 -0.1375 -0.13333333 -0.12916667 -0.125 -0.12083333 -0.11666667 -0.1125 -0.10833333 -0.10416667 -0.1 -0.09583333 -0.09166667 -0.0875 -0.08333333 -0.07916667 -0.075 -0.07083333 -0.06666667 -0.0625 -0.05833333 -0.05416667 -0.05 -0.04583333 -0.04166667 -0.0375 -0.03333333 -0.02916667 -0.025 -0.02083333 -0.01666667 -0.0125 -0.00833333 -0.00416667 0 0 0 0 0 0
  line L34 (-7.9641, 0.6184) -> (-7.9634, 0.6184)
  line L35 (-7.9634, 0.6184) -> (-7.2282, 0.5613)
  arc A18 (-7.2282, 0.5613) -> (-7.2282, -0.5613) centre (0, 0) ccw
  line L36 (-7.2282, -0.5613) -> (-7.9634, -0.6184)
  line L37 (-7.9634, -0.6184) -> (-7.9641, -0.6184)
  spline S18 degree 5 poles (-7.9641, -0.6184) (-7.9642, -0.6184) (-7.9643, -0.6184) (-7.9646, -0.6185) (-7.965, -0.6185) (-7.9656, -0.6186) (-7.9662, -0.6186) (-7.967, -0.6187) (-7.9678, -0.6188) (-7.9687, -0.6189) (-7.9697, -0.619) (-7.9708, -0.6192) (-7.972, -0.6193) (-7.9733, -0.6195) (-7.9746, -0.6196) (-7.976, -0.6198) (-7.9775, -0.62) (-7.979, -0.6202) (-7.9807, -0.6205) (-7.9824, -0.6207) (-7.9842, -0.621) (-7.9861, -0.6213) (-7.988, -0.6216) (-7.99, -0.6219) (-7.9921, -0.6222) (-7.9943, -0.6226) (-7.9965, -0.623) (-7.9988, -0.6234) (-8.0012, -0.6238) (-8.0036, -0.6242) (-8.0061, -0.6247) (-8.0087, -0.6252) (-8.0113, -0.6256) (-8.014, -0.6262) (-8.0168, -0.6267) (-8.0196, -0.6273) (-8.0225, -0.6278) (-8.0254, -0.6284) (-8.0285, -0.6291) (-8.0316, -0.6297) (-8.0347, -0.6304) (-8.0379, -0.6311) (-8.0412, -0.6318) (-8.0445, -0.6325) (-8.0479, -0.6333) (-8.0513, -0.6341) (-8.0548, -0.6349) (-8.0584, -0.6358) (-8.062, -0.6366) (-8.0656, -0.6375) (-8.0694, -0.6384) (-8.0732, -0.6394) (-8.077, -0.6403) (-8.0809, -0.6413) (-8.0848, -0.6423) (-8.0888, -0.6434) (-8.0929, -0.6444) (-8.097, -0.6455) (-8.1011, -0.6467) (-8.1053, -0.6478) (-8.1096, -0.649) (-8.1139, -0.6502) (-8.1182, -0.6514) (-8.1226, -0.6527) (-8.1271, -0.654) (-8.1316, -0.6553) (-8.1362, -0.6566) (-8.1408, -0.658) (-8.1454, -0.6594) (-8.1501, -0.6608) (-8.1548, -0.6623) (-8.1596, -0.6637) (-8.1645, -0.6653) (-8.1693, -0.6668) (-8.1743, -0.6684) (-8.1792, -0.67) (-8.1842, -0.6716) (-8.1893, -0.6733) (-8.1944, -0.675) (-8.1995, -0.6767) (-8.2047, -0.6784) (-8.2099, -0.6802) (-8.2152, -0.682) (-8.2205, -0.6839) (-8.2258, -0.6857) (-8.2312, -0.6876) (-8.2367, -0.6896) (-8.2421, -0.6915) (-8.2476, -0.6935) (-8.2532, -0.6956) (-8.2588, -0.6976) (-8.2644, -0.6997) (-8.2701, -0.7018) (-8.2758, -0.704) (-8.2815, -0.7062) (-8.2873, -0.7084) (-8.2931, -0.7106) (-8.2989, -0.7129) (-8.3048, -0.7152) (-8.3107, -0.7176) (-8.3167, -0.72) (-8.3227, -0.7224) (-8.3287, -0.7248) (-8.3348, -0.7273) (-8.3409, -0.7298) (-8.347, -0.7324) (-8.3532, -0.7349) (-8.3594, -0.7375) (-8.3656, -0.7402) (-8.3718, -0.7428) (-8.3781, -0.7456) (-8.3845, -0.7483) (-8.3908, -0.7511) (-8.3972, -0.7539) (-8.4036, -0.7567) (-8.4101, -0.7596) (-8.4166, -0.7625) (-8.4231, -0.7654) (-8.4296, -0.7684) (-8.4362, -0.7714) (-8.4428, -0.7745) (-8.4494, -0.7775) (-8.4561, -0.7807) (-8.4627, -0.7838) (-8.4695, -0.787) (-8.4762, -0.7902) (-8.483, -0.7934) (-8.4898, -0.7967) (-8.4966, -0.8) (-8.5034, -0.8034) (-8.5103, -0.8068) (-8.5172, -0.8102) (-8.5242, -0.8137) (-8.5311, -0.8172) (-8.5381, -0.8207) (-8.5451, -0.8242) (-8.5521, -0.8278) (-8.5592, -0.8315) (-8.5663, -0.8351) (-8.5734, -0.8388) (-8.5805, -0.8426) (-8.5877, -0.8463) (-8.5948, -0.8501) (-8.602, -0.854) (-8.6093, -0.8579) (-8.6165, -0.8618) (-8.6238, -0.8657) (-8.6311, -0.8697) (-8.6384, -0.8737) (-8.6457, -0.8778) (-8.6531, -0.8819) (-8.6605, -0.886) (-8.6679, -0.8902) (-8.6753, -0.8944) (-8.6827, -0.8986) (-8.6902, -0.9029) (-8.6977, -0.9072) (-8.7052, -0.9115) (-8.7127, -0.9159) (-8.7202, -0.9203) (-8.7278, -0.9247) (-8.7354, -0.9292) (-8.743, -0.9337) (-8.7506, -0.9383) (-8.7582, -0.9429) (-8.7659, -0.9475) (-8.7735, -0.9522) (-8.7812, -0.9569) (-8.7889, -0.9616) (-8.7967, -0.9664) (-8.8044, -0.9712) (-8.8122, -0.976) (-8.8199, -0.9809) (-8.8277, -0.9858) (-8.8355, -0.9908) (-8.8434, -0.9958) (-8.8512, -1.0008) (-8.8591, -1.0059) (-8.8669, -1.011) (-8.8748, -1.0161) (-8.8827, -1.0213) (-8.8906, -1.0265) (-8.8986, -1.0317) (-8.9065, -1.037) (-8.9145, -1.0423) (-8.9225, -1.0477) (-8.9305, -1.0531) (-8.9385, -1.0585) (-8.9465, -1.0639) (-8.9545, -1.0694) (-8.9625, -1.075) (-8.9706, -1.0805) (-8.9787, -1.0862) (-8.9867, -1.0918) (-8.9948, -1.0975) (-9.0029, -1.1032) (-9.0111, -1.109) (-9.0192, -1.1147) (-9.0273, -1.1206) (-9.0355, -1.1264) (-9.0436, -1.1323) (-9.0518, -1.1383) (-9.06, -1.1443) (-9.0682, -1.1503) (-9.0764, -1.1563) (-9.0846, -1.1624) (-9.0929, -1.1685) (-9.1011, -1.1747) (-9.1093, -1.1809) (-9.1176, -1.1871) (-9.1259, -1.1934) (-9.1341, -1.1997) (-9.1424, -1.206) (-9.1507, -1.2124) (-9.159, -1.2188) (-9.1673, -1.2253) (-9.1756, -1.2317) (-9.184, -1.2383) (-9.1923, -1.2448) (-9.2006, -1.2514) (-9.209, -1.2581) (-9.2173, -1.2647) (-9.2257, -1.2714) (-9.2341, -1.2782) (-9.2425, -1.285) (-9.2508, -1.2918) (-9.2592, -1.2986) (-9.2676, -1.3055) (-9.276, -1.3125) (-9.2845, -1.3194) (-9.2929, -1.3264) (-9.3013, -1.3335) (-9.3097, -1.3405) (-9.3182, -1.3476) (-9.3266, -1.3548) (-9.335, -1.362) (-9.3435, -1.3692) (-9.3519, -1.3765) (-9.3604, -1.3837) (-9.3689, -1.3911) (-9.3773, -1.3984) (-9.3841, -1.4044) (-9.3892, -1.4088) (-9.3926, -1.4118) (-9.3943, -1.4133) knots 0 0 0 0 0 0 0.00416667 0.00833333 0.0125 0.01666667 0.02083333 0.025 0.02916667 0.03333333 0.0375 0.04166667 0.04583333 0.05 0.05416667 0.05833333 0.0625 0.06666667 0.07083333 0.075 0.07916667 0.08333333 0.0875 0.09166667 0.09583333 0.1 0.10416667 0.10833333 0.1125 0.11666667 0.12083333 0.125 0.12916667 0.13333333 0.1375 0.14166667 0.14583333 0.15 0.15416667 0.15833333 0.1625 0.16666667 0.17083333 0.175 0.17916667 0.18333333 0.1875 0.19166667 0.19583333 0.2 0.20416667 0.20833333 0.2125 0.21666667 0.22083333 0.225 0.22916667 0.23333333 0.2375 0.24166667 0.24583333 0.25 0.25416667 0.25833333 0.2625 0.26666667 0.27083333 0.275 0.27916667 0.28333333 0.2875 0.29166667 0.29583333 0.3 0.30416667 0.30833333 0.3125 0.31666667 0.32083333 0.325 0.32916667 0.33333333 0.3375 0.34166667 0.34583333 0.35 0.35416667 0.35833333 0.3625 0.36666667 0.37083333 0.375 0.37916667 0.38333333 0.3875 0.39166667 0.39583333 0.4 0.40416667 0.40833333 0.4125 0.41666667 0.42083333 0.425 0.42916667 0.43333333 0.4375 0.44166667 0.44583333 0.45 0.45416667 0.45833333 0.4625 0.46666667 0.47083333 0.475 0.47916667 0.48333333 0.4875 0.49166667 0.49583333 0.5 0.50416667 0.50833333 0.5125 0.51666667 0.52083333 0.525 0.52916667 0.53333333 0.5375 0.54166667 0.54583333 0.55 0.55416667 0.55833333 0.5625 0.56666667 0.57083333 0.575 0.57916667 0.58333333 0.5875 0.59166667 0.59583333 0.6 0.60416667 0.60833333 0.6125 0.61666667 0.62083333 0.625 0.62916667 0.63333333 0.6375 0.64166667 0.64583333 0.65 0.65416667 0.65833333 0.6625 0.66666667 0.67083333 0.675 0.67916667 0.68333333 0.6875 0.69166667 0.69583333 0.7 0.70416667 0.70833333 0.7125 0.71666667 0.72083333 0.725 0.72916667 0.73333333 0.7375 0.74166667 0.74583333 0.75 0.75416667 0.75833333 0.7625 0.76666667 0.77083333 0.775 0.77916667 0.78333333 0.7875 0.79166667 0.79583333 0.8 0.80416667 0.80833333 0.8125 0.81666667 0.82083333 0.825 0.82916667 0.83333333 0.8375 0.84166667 0.84583333 0.85 0.85416667 0.85833333 0.8625 0.86666667 0.87083333 0.875 0.87916667 0.88333333 0.8875 0.89166667 0.89583333 0.9 0.90416667 0.90833333 0.9125 0.91666667 0.92083333 0.925 0.92916667 0.93333333 0.9375 0.94166667 0.94583333 0.95 0.95416667 0.95833333 0.9625 0.96666667 0.97083333 0.975 0.97916667 0.98333333 0.9875 0.99166667 0.99583333 1 1 1 1 1 1
  arc A19 (-9.3943, -1.4133) -> (-9.2705, -2.0758) centre (0, 0) ccw
  spline S19 degree 5 poles (-9.2705, -2.0758) (-9.2683, -2.0765) (-9.2641, -2.0781) (-9.2577, -2.0804) (-9.2493, -2.0835) (-9.2387, -2.0873) (-9.2282, -2.0911) (-9.2177, -2.0948) (-9.2072, -2.0985) (-9.1967, -2.1022) (-9.1862, -2.1058) (-9.1757, -2.1095) (-9.1653, -2.113) (-9.1549, -2.1166) (-9.1445, -2.1201) (-9.1341, -2.1236) (-9.1238, -2.1271) (-9.1134, -2.1305) (-9.1031, -2.1339) (-9.0928, -2.1372) (-9.0825, -2.1406) (-9.0723, -2.1439) (-9.062, -2.1471) (-9.0518, -2.1504) (-9.0416, -2.1536) (-9.0314, -2.1567) (-9.0212, -2.1599) (-9.0111, -2.163) (-9.001, -2.1661) (-8.9909, -2.1691) (-8.9808, -2.1721) (-8.9707, -2.1751) (-8.9607, -2.178) (-8.9507, -2.181) (-8.9407, -2.1839) (-8.9307, -2.1867) (-8.9208, -2.1895) (-8.9109, -2.1923) (-8.9009, -2.1951) (-8.8911, -2.1978) (-8.8812, -2.2005) (-8.8714, -2.2032) (-8.8616, -2.2059) (-8.8518, -2.2085) (-8.842, -2.2111) (-8.8323, -2.2136) (-8.8225, -2.2161) (-8.8128, -2.2186) (-8.8032, -2.2211) (-8.7935, -2.2235) (-8.7839, -2.2259) (-8.7743, -2.2283) (-8.7647, -2.2307) (-8.7552, -2.233) (-8.7456, -2.2353) (-8.7361, -2.2375) (-8.7267, -2.2397) (-8.7172, -2.2419) (-8.7078, -2.2441) (-8.6984, -2.2463) (-8.689, -2.2484) (-8.6797, -2.2504) (-8.6704, -2.2525) (-8.6611, -2.2545) (-8.6518, -2.2565) (-8.6426, -2.2585) (-8.6334, -2.2604) (-8.6242, -2.2623) (-8.615, -2.2642) (-8.6059, -2.2661) (-8.5968, -2.2679) (-8.5877, -2.2697) (-8.5787, -2.2715) (-8.5697, -2.2732) (-8.5607, -2.2749) (-8.5517, -2.2766) (-8.5428, -2.2783) (-8.5339, -2.2799) (-8.5251, -2.2815) (-8.5162, -2.2831) (-8.5074, -2.2846) (-8.4986, -2.2861) (-8.4899, -2.2876) (-8.4812, -2.2891) (-8.4725, -2.2906) (-8.4638, -2.292) (-8.4552, -2.2934) (-8.4466, -2.2947) (-8.438, -2.2961) (-8.4295, -2.2974) (-8.421, -2.2986) (-8.4125, -2.2999) (-8.4041, -2.3011) (-8.3957, -2.3023) (-8.3873, -2.3035) (-8.379, -2.3047) (-8.3707, -2.3058) (-8.3624, -2.3069) (-8.3542, -2.308) (-8.346, -2.3091) (-8.3378, -2.3101) (-8.3297, -2.3111) (-8.3216, -2.3121) (-8.3135, -2.313) (-8.3055, -2.314) (-8.2975, -2.3149) (-8.2895, -2.3158) (-8.2816, -2.3166) (-8.2737, -2.3174) (-8.2658, -2.3183) (-8.258, -2.3191) (-8.2502, -2.3198) (-8.2425, -2.3206) (-8.2348, -2.3213) (-8.2271, -2.322) (-8.2194, -2.3226) (-8.2118, -2.3233) (-8.2043, -2.3239) (-8.1968, -2.3245) (-8.1893, -2.3251) (-8.1818, -2.3257) (-8.1744, -2.3262) (-8.167, -2.3267) (-8.1597, -2.3272) (-8.1524, -2.3277) (-8.1452, -2.3282) (-8.138, -2.3286) (-8.1308, -2.329) (-8.1236, -2.3294) (-8.1166, -2.3298) (-8.1095, -2.3301) (-8.1025, -2.3305) (-8.0955, -2.3308) (-8.0886, -2.3311) (-8.0817, -2.3313) (-8.0749, -2.3316) (-8.0681, -2.3318) (-8.0613, -2.332) (-8.0546, -2.3322) (-8.0479, -2.3324) (-8.0413, -2.3325) (-8.0347, -2.3327) (-8.0281, -2.3328) (-8.0216, -2.3329) (-8.0152, -2.333) (-8.0088, -2.3331) (-8.0024, -2.3331) (-7.9961, -2.3331) (-7.9898, -2.3331) (-7.9836, -2.3331) (-7.9774, -2.3331) (-7.9712, -2.3331) (-7.9651, -2.333) (-7.9591, -2.333) (-7.9531, -2.3329) (-7.9471, -2.3328) (-7.9412, -2.3327) (-7.9354, -2.3326) (-7.9296, -2.3324) (-7.9238, -2.3323) (-7.9181, -2.3321) (-7.9124, -2.3319) (-7.9068, -2.3317) (-7.9012, -2.3315) (-7.8957, -2.3313) (-7.8903, -2.331) (-7.8849, -2.3308) (-7.8795, -2.3305) (-7.8742, -2.3302) (-7.8689, -2.3299) (-7.8637, -2.3296) (-7.8586, -2.3293) (-7.8534, -2.329) (-7.8484, -2.3287) (-7.8434, -2.3283) (-7.8384, -2.328) (-7.8336, -2.3276) (-7.8287, -2.3272) (-7.8239, -2.3268) (-7.8192, -2.3265) (-7.8145, -2.3261) (-7.8099, -2.3256) (-7.8054, -2.3252) (-7.8008, -2.3248) (-7.7964, -2.3244) (-7.792, -2.3239) (-7.7877, -2.3235) (-7.7834, -2.323) (-7.7792, -2.3226) (-7.775, -2.3221) (-7.7709, -2.3216) (-7.7669, -2.3211) (-7.7629, -2.3207) (-7.759, -2.3202) (-7.7551, -2.3197) (-7.7513, -2.3192) (-7.7475, -2.3187) (-7.7439, -2.3182) (-7.7402, -2.3177) (-7.7367, -2.3172) (-7.7332, -2.3167) (-7.7298, -2.3162) (-7.7264, -2.3157) (-7.7231, -2.3151) (-7.7199, -2.3146) (-7.7167, -2.3141) (-7.7136, -2.3136) (-7.7105, -2.3131) (-7.7076, -2.3126) (-7.7046, -2.3121) (-7.7018, -2.3116) (-7.699, -2.3111) (-7.6963, -2.3106) (-7.6937, -2.3101) (-7.6911, -2.3096) (-7.6886, -2.3092) (-7.6862, -2.3087) (-7.6838, -2.3082) (-7.6816, -2.3078) (-7.6793, -2.3073) (-7.6772, -2.3069) (-7.6751, -2.3064) (-7.6731, -2.306) (-7.6712, -2.3056) (-7.6694, -2.3052) (-7.6676, -2.3048) (-7.6659, -2.3044) (-7.6643, -2.304) (-7.6628, -2.3036) (-7.6613, -2.3033) (-7.6599, -2.303) (-7.6586, -2.3026) (-7.6574, -2.3023) (-7.6562, -2.302) (-7.6552, -2.3018) (-7.6542, -2.3015) (-7.6533, -2.3013) (-7.6525, -2.3011) (-7.6518, -2.3009) (-7.6511, -2.3007) (-7.6505, -2.3005) (-7.6502, -2.3004) (-7.6499, -2.3004) (-7.6498, -2.3003) (-7.6497, -2.3003) knots -1 -1 -1 -1 -1 -1 -0.99583333 -0.99166667 -0.9875 -0.98333333 -0.97916667 -0.975 -0.97083333 -0.96666667 -0.9625 -0.95833333 -0.95416667 -0.95 -0.94583333 -0.94166667 -0.9375 -0.93333333 -0.92916667 -0.925 -0.92083333 -0.91666667 -0.9125 -0.90833333 -0.90416667 -0.9 -0.89583333 -0.89166667 -0.8875 -0.88333333 -0.87916667 -0.875 -0.87083333 -0.86666667 -0.8625 -0.85833333 -0.85416667 -0.85 -0.84583333 -0.84166667 -0.8375 -0.83333333 -0.82916667 -0.825 -0.82083333 -0.81666667 -0.8125 -0.80833333 -0.80416667 -0.8 -0.79583333 -0.79166667 -0.7875 -0.78333333 -0.77916667 -0.775 -0.77083333 -0.76666667 -0.7625 -0.75833333 -0.75416667 -0.75 -0.74583333 -0.74166667 -0.7375 -0.73333333 -0.72916667 -0.725 -0.72083333 -0.71666667 -0.7125 -0.70833333 -0.70416667 -0.7 -0.69583333 -0.69166667 -0.6875 -0.68333333 -0.67916667 -0.675 -0.67083333 -0.66666667 -0.6625 -0.65833333 -0.65416667 -0.65 -0.64583333 -0.64166667 -0.6375 -0.63333333 -0.62916667 -0.625 -0.62083333 -0.61666667 -0.6125 -0.60833333 -0.60416667 -0.6 -0.59583333 -0.59166667 -0.5875 -0.58333333 -0.57916667 -0.575 -0.57083333 -0.56666667 -0.5625 -0.55833333 -0.55416667 -0.55 -0.54583333 -0.54166667 -0.5375 -0.53333333 -0.52916667 -0.525 -0.52083333 -0.51666667 -0.5125 -0.50833333 -0.50416667 -0.5 -0.49583333 -0.49166667 -0.4875 -0.48333333 -0.47916667 -0.475 -0.47083333 -0.46666667 -0.4625 -0.45833333 -0.45416667 -0.45 -0.44583333 -0.44166667 -0.4375 -0.43333333 -0.42916667 -0.425 -0.42083333 -0.41666667 -0.4125 -0.40833333 -0.40416667 -0.4 -0.39583333 -0.39166667 -0.3875 -0.38333333 -0.37916667 -0.375 -0.37083333 -0.36666667 -0.3625 -0.35833333 -0.35416667 -0.35 -0.34583333 -0.34166667 -0.3375 -0.33333333 -0.32916667 -0.325 -0.32083333 -0.31666667 -0.3125 -0.30833333 -0.30416667 -0.3 -0.29583333 -0.29166667 -0.2875 -0.28333333 -0.27916667 -0.275 -0.27083333 -0.26666667 -0.2625 -0.25833333 -0.25416667 -0.25 -0.24583333 -0.24166667 -0.2375 -0.23333333 -0.22916667 -0.225 -0.22083333 -0.21666667 -0.2125 -0.20833333 -0.20416667 -0.2 -0.19583333 -0.19166667 -0.1875 -0.18333333 -0.17916667 -0.175 -0.17083333 -0.16666667 -0.1625 -0.15833333 -0.15416667 -0.15 -0.14583333 -0.14166667 -0.1375 -0.13333333 -0.12916667 -0.125 -0.12083333 -0.11666667 -0.1125 -0.10833333 -0.10416667 -0.1 -0.09583333 -0.09166667 -0.0875 -0.08333333 -0.07916667 -0.075 -0.07083333 -0.06666667 -0.0625 -0.05833333 -0.05416667 -0.05 -0.04583333 -0.04166667 -0.0375 -0.03333333 -0.02916667 -0.025 -0.02083333 -0.01666667 -0.0125 -0.00833333 -0.00416667 0 0 0 0 0 0
  line L38 (-7.6497, -2.3003) -> (-7.649, -2.3001)
  line L39 (-7.649, -2.3001) -> (-6.9429, -2.0878)
  arc A20 (-6.9429, -2.0878) -> (-6.5374, -3.1345) centre (0, 0) ccw
  line L40 (-6.5374, -3.1345) -> (-7.2023, -3.4533)
  line L41 (-7.2023, -3.4533) -> (-7.2029, -3.4536)
  spline S20 degree 5 poles (-7.2029, -3.4536) (-7.203, -3.4537) (-7.2031, -3.4537) (-7.2033, -3.4538) (-7.2037, -3.454) (-7.2042, -3.4543) (-7.2048, -3.4546) (-7.2055, -3.4549) (-7.2062, -3.4553) (-7.207, -3.4558) (-7.2079, -3.4562) (-7.2089, -3.4567) (-7.21, -3.4573) (-7.2111, -3.4579) (-7.2122, -3.4585) (-7.2135, -3.4592) (-7.2148, -3.46) (-7.2162, -3.4607) (-7.2176, -3.4615) (-7.2191, -3.4624) (-7.2207, -3.4633) (-7.2224, -3.4642) (-7.2241, -3.4652) (-7.2258, -3.4662) (-7.2276, -3.4673) (-7.2295, -3.4684) (-7.2315, -3.4696) (-7.2335, -3.4708) (-7.2355, -3.472) (-7.2376, -3.4733) (-7.2398, -3.4746) (-7.242, -3.476) (-7.2443, -3.4774) (-7.2466, -3.4789) (-7.249, -3.4804) (-7.2515, -3.4819) (-7.2539, -3.4835) (-7.2565, -3.4851) (-7.2591, -3.4868) (-7.2617, -3.4885) (-7.2644, -3.4903) (-7.2671, -3.4921) (-7.2699, -3.4939) (-7.2728, -3.4958) (-7.2756, -3.4978) (-7.2786, -3.4998) (-7.2815, -3.5018) (-7.2845, -3.5038) (-7.2876, -3.506) (-7.2907, -3.5081) (-7.2938, -3.5103) (-7.297, -3.5125) (-7.3003, -3.5148) (-7.3035, -3.5172) (-7.3068, -3.5195) (-7.3102, -3.5219) (-7.3136, -3.5244) (-7.317, -3.5269) (-7.3205, -3.5295) (-7.324, -3.532) (-7.3275, -3.5347) (-7.3311, -3.5374) (-7.3347, -3.5401) (-7.3384, -3.5428) (-7.3421, -3.5456) (-7.3458, -3.5485) (-7.3495, -3.5514) (-7.3533, -3.5543) (-7.3572, -3.5573) (-7.361, -3.5603) (-7.3649, -3.5634) (-7.3688, -3.5665) (-7.3728, -3.5697) (-7.3768, -3.5729) (-7.3808, -3.5761) (-7.3849, -3.5794) (-7.389, -3.5827) (-7.3931, -3.5861) (-7.3972, -3.5895) (-7.4014, -3.593) (-7.4056, -3.5965) (-7.4098, -3.6) (-7.4141, -3.6036) (-7.4183, -3.6073) (-7.4227, -3.611) (-7.427, -3.6147) (-7.4314, -3.6184) (-7.4357, -3.6222) (-7.4402, -3.6261) (-7.4446, -3.63) (-7.4491, -3.6339) (-7.4536, -3.6379) (-7.4581, -3.6419) (-7.4626, -3.646) (-7.4672, -3.6501) (-7.4718, -3.6543) (-7.4764, -3.6585) (-7.481, -3.6627) (-7.4856, -3.667) (-7.4903, -3.6713) (-7.495, -3.6757) (-7.4997, -3.6801) (-7.5045, -3.6846) (-7.5092, -3.6891) (-7.514, -3.6936) (-7.5188, -3.6982) (-7.5236, -3.7028) (-7.5284, -3.7075) (-7.5333, -3.7122) (-7.5382, -3.7169) (-7.5431, -3.7217) (-7.548, -3.7266) (-7.5529, -3.7315) (-7.5578, -3.7364) (-7.5628, -3.7414) (-7.5678, -3.7464) (-7.5728, -3.7514) (-7.5778, -3.7565) (-7.5828, -3.7616) (-7.5878, -3.7668) (-7.5929, -3.7721) (-7.5979, -3.7773) (-7.603, -3.7826) (-7.6081, -3.788) (-7.6132, -3.7934) (-7.6184, -3.7988) (-7.6235, -3.8043) (-7.6287, -3.8098) (-7.6338, -3.8153) (-7.639, -3.8209) (-7.6442, -3.8266) (-7.6494, -3.8323) (-7.6546, -3.838) (-7.6598, -3.8438) (-7.6651, -3.8496) (-7.6703, -3.8554) (-7.6756, -3.8613) (-7.6808, -3.8673) (-7.6861, -3.8732) (-7.6914, -3.8793) (-7.6967, -3.8853) (-7.702, -3.8914) (-7.7073, -3.8976) (-7.7127, -3.9037) (-7.718, -3.91) (-7.7233, -3.9162) (-7.7287, -3.9225) (-7.7341, -3.9289) (-7.7394, -3.9353) (-7.7448, -3.9417) (-7.7502, -3.9482) (-7.7556, -3.9547) (-7.761, -3.9612) (-7.7664, -3.9678) (-7.7718, -3.9745) (-7.7772, -3.9811) (-7.7826, -3.9879) (-7.788, -3.9946) (-7.7935, -4.0014) (-7.7989, -4.0082) (-7.8044, -4.0151) (-7.8098, -4.022) (-7.8153, -4.029) (-7.8207, -4.036) (-7.8262, -4.043) (-7.8317, -4.0501) (-7.8371, -4.0572) (-7.8426, -4.0644) (-7.8481, -4.0716) (-7.8536, -4.0788) (-7.859, -4.0861) (-7.8645, -4.0934) (-7.87, -4.1008) (-7.8755, -4.1082) (-7.881, -4.1156) (-7.8865, -4.1231) (-7.892, -4.1306) (-7.8975, -4.1382) (-7.903, -4.1458) (-7.9085, -4.1534) (-7.914, -4.1611) (-7.9195, -4.1688) (-7.925, -4.1766) (-7.9305, -4.1844) (-7.936, -4.1922) (-7.9415, -4.2001) (-7.947, -4.208) (-7.9525, -4.2159) (-7.958, -4.2239) (-7.9635, -4.232) (-7.969, -4.24) (-7.9745, -4.2481) (-7.98, -4.2563) (-7.9855, -4.2645) (-7.991, -4.2727) (-7.9965, -4.2809) (-8.002, -4.2892) (-8.0075, -4.2976) (-8.0129, -4.306) (-8.0184, -4.3144) (-8.0239, -4.3228) (-8.0294, -4.3313) (-8.0349, -4.3398) (-8.0403, -4.3484) (-8.0458, -4.357) (-8.0513, -4.3656) (-8.0567, -4.3743) (-8.0622, -4.383) (-8.0676, -4.3918) (-8.0731, -4.4006) (-8.0785, -4.4094) (-8.084, -4.4183) (-8.0894, -4.4272) (-8.0948, -4.4361) (-8.1002, -4.4451) (-8.1057, -4.4541) (-8.1111, -4.4632) (-8.1165, -4.4723) (-8.1219, -4.4814) (-8.1273, -4.4906) (-8.1327, -4.4998) (-8.138, -4.509) (-8.1434, -4.5183) (-8.1488, -4.5276) (-8.1542, -4.537) (-8.1595, -4.5463) (-8.1649, -4.5558) (-8.1702, -4.5652) (-8.1755, -4.5747) (-8.1809, -4.5843) (-8.1862, -4.5938) (-8.1915, -4.6034) (-8.1968, -4.6131) (-8.2021, -4.6227) (-8.2074, -4.6325) (-8.2127, -4.6422) (-8.2179, -4.652) (-8.2232, -4.6618) (-8.2284, -4.6717) (-8.2337, -4.6816) (-8.2389, -4.6915) (-8.2431, -4.6995) (-8.2462, -4.7055) (-8.2483, -4.7095) (-8.2494, -4.7115) knots 0 0 0 0 0 0 0.00416667 0.00833333 0.0125 0.01666667 0.02083333 0.025 0.02916667 0.03333333 0.0375 0.04166667 0.04583333 0.05 0.05416667 0.05833333 0.0625 0.06666667 0.07083333 0.075 0.07916667 0.08333333 0.0875 0.09166667 0.09583333 0.1 0.10416667 0.10833333 0.1125 0.11666667 0.12083333 0.125 0.12916667 0.13333333 0.1375 0.14166667 0.14583333 0.15 0.15416667 0.15833333 0.1625 0.16666667 0.17083333 0.175 0.17916667 0.18333333 0.1875 0.19166667 0.19583333 0.2 0.20416667 0.20833333 0.2125 0.21666667 0.22083333 0.225 0.22916667 0.23333333 0.2375 0.24166667 0.24583333 0.25 0.25416667 0.25833333 0.2625 0.26666667 0.27083333 0.275 0.27916667 0.28333333 0.2875 0.29166667 0.29583333 0.3 0.30416667 0.30833333 0.3125 0.31666667 0.32083333 0.325 0.32916667 0.33333333 0.3375 0.34166667 0.34583333 0.35 0.35416667 0.35833333 0.3625 0.36666667 0.37083333 0.375 0.37916667 0.38333333 0.3875 0.39166667 0.39583333 0.4 0.40416667 0.40833333 0.4125 0.41666667 0.42083333 0.425 0.42916667 0.43333333 0.4375 0.44166667 0.44583333 0.45 0.45416667 0.45833333 0.4625 0.46666667 0.47083333 0.475 0.47916667 0.48333333 0.4875 0.49166667 0.49583333 0.5 0.50416667 0.50833333 0.5125 0.51666667 0.52083333 0.525 0.52916667 0.53333333 0.5375 0.54166667 0.54583333 0.55 0.55416667 0.55833333 0.5625 0.56666667 0.57083333 0.575 0.57916667 0.58333333 0.5875 0.59166667 0.59583333 0.6 0.60416667 0.60833333 0.6125 0.61666667 0.62083333 0.625 0.62916667 0.63333333 0.6375 0.64166667 0.64583333 0.65 0.65416667 0.65833333 0.6625 0.66666667 0.67083333 0.675 0.67916667 0.68333333 0.6875 0.69166667 0.69583333 0.7 0.70416667 0.70833333 0.7125 0.71666667 0.72083333 0.725 0.72916667 0.73333333 0.7375 0.74166667 0.74583333 0.75 0.75416667 0.75833333 0.7625 0.76666667 0.77083333 0.775 0.77916667 0.78333333 0.7875 0.79166667 0.79583333 0.8 0.80416667 0.80833333 0.8125 0.81666667 0.82083333 0.825 0.82916667 0.83333333 0.8375 0.84166667 0.84583333 0.85 0.85416667 0.85833333 0.8625 0.86666667 0.87083333 0.875 0.87916667 0.88333333 0.8875 0.89166667 0.89583333 0.9 0.90416667 0.90833333 0.9125 0.91666667 0.92083333 0.925 0.92916667 0.93333333 0.9375 0.94166667 0.94583333 0.95 0.95416667 0.95833333 0.9625 0.96666667 0.97083333 0.975 0.97916667 0.98333333 0.9875 0.99166667 0.99583333 1 1 1 1 1 1
  arc A21 (-8.2494, -4.7115) -> (-7.8946, -5.2845) centre (0, 0) ccw